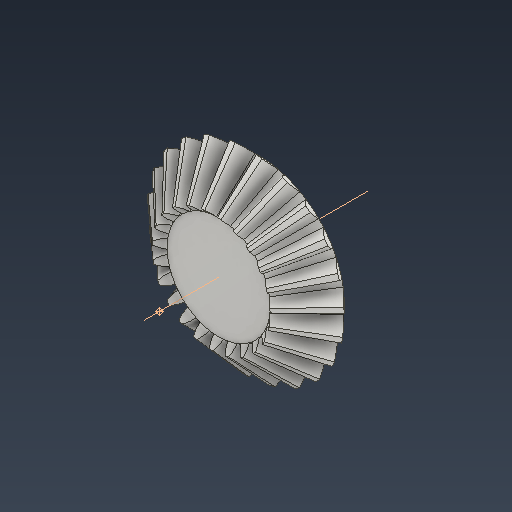
# Autodesk Inventor part: Kegelrad1
Saved by Autodesk Inventor 2021 (Build 250183000, 183)
## iProperties
Created: 2021-01-24
Part Number: Kegelrad1
Material: Steel, Mild
Document SubType Name: Modeling
Designer: laure
Categories: <?xml version="1.0" encoding="UTF-16"?> <MemberInstance><Categories><FamilyTemplate><FamilyTemplateParameter ValueType="xs:double" Id="1" ObjectReferenceKey="da_z" ObjectType="kUserParameterObject"/><FamilyTemplateParameter ValueType="xs:double" Id="2" ObjectReferenceKey="da_b" ObjectType="kUserParameterObject"/><FamilyTemplateParameter ValueType="xs:double" Id="3" ObjectReferenceKey="da_beta" ObjectType="kUserParameterObject"/><FamilyTemplateParameter ValueType="xs:double" Id="4" ObjectReferenceKey="da_dae" ObjectType="kUserParameterObject"/><FamilyTemplateParameter ValueType="xs:double" Id="5" ObjectReferenceKey="da_ve" ObjectType="kUserParameterObject"/><FamilyTemplateParameter ValueType="xs:double" Id="6" ObjectReferenceKey="da_omega" ObjectType="kUserParameterObject"/><FamilyTemplateParameter ValueType="xs:string" Id="7" ObjectReferenceKey="EAIAABAAAAAAHwAAAAAAAIAAAAAAAAAA" ObjectType="83914240" SubObjectId="SurfaceGeometry"/></FamilyTemplate><ParamToTemplateMap><ParamToTemplate CategoryParameter="//CategoryParameter[@InternalName='046C89C9-8512-4d59-83FE-43B91F4F132A']" TemplateParameter="1"/><ParamToTemplate CategoryParameter="//CategoryParameter[@InternalName='2552DF32-E462-4b46-AEBF-C6C7768E72AC']" TemplateParameter="2"/><ParamToTemplate CategoryParameter="//CategoryParameter[@InternalName='C9EE641D-15FC-4fae-A226-E94C4372FDD7']" TemplateParameter="3"/><ParamToTemplate><ParamToTemplate CategoryParameter="//CategoryParameter[@InternalName='00B6519A-459B-49c7-AD84-2E56D39A5744']" ConstantValue="0.000000"/></ParamToTemplate><ParamToTemplate><ParamToTemplate CategoryParameter="//CategoryParameter[@InternalName='04B31F0E-C7A6-4894-AA32-9629BEFACF47']" ConstantValue="1.000000"/></ParamToTemplate><ParamToTemplate><ParamToTemplate CategoryParameter="//CategoryParameter[@InternalName='43CBEC2E-7847-49e7-A936-2F7889FCB2D9']" ConstantValue="0.200000"/></ParamToTemplate><ParamToTemplate><ParamToTemplate CategoryParameter="//CategoryParameter[@InternalName='B1EFC894-105D-4ebd-86BF-FA20ED196853']" ConstantValue="0.300000"/></ParamToTemplate><ParamToTemplate><ParamToTemplate CategoryParameter="//CategoryParameter[@InternalName='51175063-3D10-4879-93E8-6246FE8B403D']" ConstantValue="2060000000.000000"/></ParamToTemplate><ParamToTemplate><ParamToTemplate CategoryParameter="//CategoryParameter[@InternalName='A3A52E27-4454-46a9-B0BD-C932399B70AF']" ConstantValue="0.300000"/></ParamToTemplate><ParamToTemplate CategoryParameter="//CategoryParameter[@InternalName='2A200944-5A8C-41ca-B96E-8520D2E510F1']" TemplateParameter="4"/><ParamToTemplate><ParamToTemplate CategoryParameter="//CategoryParameter[@InternalName='1A637F62-92C8-44bc-B81F-10802510B579']" ConstantValue="2.931322"/></ParamToTemplate><ParamToTemplate CategoryParameter="//CategoryParameter[@InternalName='B52DD4BE-6863-48fb-BF58-89EF6F9EC65C']" TemplateParameter="5"/><ParamToTemplate><ParamToTemplate CategoryParameter="//CategoryParameter[@InternalName='3956BFF2-84D2-457d-93C2-9B0613DEBA67']" ConstantValue="1.295862"/></ParamToTemplate><ParamToTemplate CategoryParameter="//CategoryParameter[@InternalName='739CFA02-461B-4bf8-8049-181FCAD8B28F']" TemplateParameter="6"/><ParamToTemplate><ParamToTemplate CategoryParameter="//CategoryParameter[@InternalName='A27E999F-E2CE-4481-8A2A-EBF499C4C3C5']" ConstantValue="0.000000"/></ParamToTemplate><ParamToTemplate><ParamToTemplate CategoryParameter="//CategoryParameter[@InternalName='9E1B4470-B2D3-4ff1-B813-535BB4CDF51A']" ConstantValue="3520000.000000"/></ParamToTemplate><ParamToTemplate><ParamToTemplate CategoryParameter="//CategoryParameter[@InternalName='F8452263-BFF6-458c-9FB1-07C4B99E95CD']" ConstantValue="11400000.000000"/></ParamToTemplate><ParamToTemplate><ParamToTemplate CategoryParameter="//CategoryParameter[@InternalName='3E3BB259-FD49-497f-8171-6EBC954A3479']" ConstantValue="2.000000"/></ParamToTemplate><ParamToTemplate CategoryParameter="//CategoryParameter[@InternalName='27C3BAF2-7550-4e4b-AE2C-0DB134B7D9B7']" TemplateParameter="7"/></ParamToTemplateMap><Category DisplayName="Gear" InternalName="DC85795E-93AB-48d5-8EEE-5A27447B64BD" Mnemonic="Gear"><CategoryParameter DisplayName="z" InternalName="046C89C9-8512-4d59-83FE-43B91F4F132A" Mnemonic="z"/><CategoryParameter DisplayName="b" InternalName="2552DF32-E462-4b46-AEBF-C6C7768E72AC" Mnemonic="b"/><CategoryParameter DisplayName="||b|" InternalName="C9EE641D-15FC-4fae-A226-E94C4372FDD7" Mnemonic="beta"/><CategoryParameter DisplayName="x" InternalName="00B6519A-459B-49c7-AD84-2E56D39A5744" Mnemonic="x"/><CategoryParameter DisplayName="a*" InternalName="04B31F0E-C7A6-4894-AA32-9629BEFACF47" Mnemonic="a"/><CategoryParameter DisplayName="c*" InternalName="43CBEC2E-7847-49e7-A936-2F7889FCB2D9" Mnemonic="c"/><CategoryParameter DisplayName="r|.f|*" InternalName="B1EFC894-105D-4ebd-86BF-FA20ED196853" Mnemonic="rf"/><CategoryParameter DisplayName="E" InternalName="51175063-3D10-4879-93E8-6246FE8B403D" Mnemonic="E"/><CategoryParameter DisplayName="||m|" InternalName="A3A52E27-4454-46a9-B0BD-C932399B70AF" Mnemonic="mi"/><Category DisplayName="BevelGear" InternalName="0C98F69A-0C2B-4791-B2FE-7691BB227E77" Mnemonic="BevelGear"><CategoryParameter DisplayName="d|.ae|" InternalName="2A200944-5A8C-41ca-B96E-8520D2E510F1" Mnemonic="dae"/><CategoryParameter DisplayName="d|.ai|" InternalName="1A637F62-92C8-44bc-B81F-10802510B579" Mnemonic="dai"/><CategoryParameter DisplayName="A|.e|" InternalName="B52DD4BE-6863-48fb-BF58-89EF6F9EC65C" Mnemonic="ve"/><CategoryParameter DisplayName="A|.i|" InternalName="3956BFF2-84D2-457d-93C2-9B0613DEBA67" Mnemonic="vi"/><CategoryParameter DisplayName="||S|" InternalName="739CFA02-461B-4bf8-8049-181FCAD8B28F" Mnemonic="omega"/><CategoryParameter DisplayName="x|.t|" InternalName="A27E999F-E2CE-4481-8A2A-EBF499C4C3C5" Mnemonic="xt"/><CategoryParameter DisplayName="||s||.Flim|" InternalName="9E1B4470-B2D3-4ff1-B813-535BB4CDF51A" Mnemonic="sFlim"/><CategoryParameter DisplayName="||s||.Hlim|" InternalName="F8452263-BFF6-458c-9FB1-07C4B99E95CD" Mnemonic="sHlim"/><CategoryParameter DisplayName="Typ" InternalName="3E3BB259-FD49-497f-8171-6EBC954A3479" Mnemonic="type"/><CategoryParameter DisplayName="PitchDiameter" InternalName="27C3BAF2-7550-4e4b-AE2C-0DB134B7D9B7" Mnemonic="IDS_PITCHDIAM"/></Category></Category></Categories></MemberInstance>
Mass: 60.9118 g
Surface Area: 34.3074 cm^2
Volume: 7.7496 cm^3
Density: 7.86 g/cm^3
Appearance: Steel
CustomPartVersion: 1
Author: laure
Autodesk Inventor part; units mm, degrees
ref_plane "Netzebene2" through (0, 0, 0) normal (0.9906859, 0.1361666, 0) x (0, 0, 1)
sketch "Skizze des Zahnradkörpers" plane through (0, 0, 0) normal (1, 0, 0) x (0, 1, 0)
  line L0 (0, 0) -> (21.302944, -24.697056) construction
  line L1 (21.302944, -24.697056) -> (24.414214, -21.585786)
  line L2 (24.414214, -21.585786) -> (0, 0) construction
  line L3 (23, -23) -> (0, 0) construction
  line L4 (12.788816, -14.826407) -> (14.656608, -12.958616)
  line L5 (21.302944, -24.697056) -> (12.788816, -14.826407)
  line L6 (24.414214, -21.585786) -> (14.656608, -12.958616)
  line L7 (0, -39.386751) -> (0, 6.564458)
  line L8 (0, -23) -> (24.414214, -23) construction
  dimension "d0" = 46
  dimension "d1" = 42.60589
  dimension "d2" = 48.82843
  dimension "d3" = 13
  dimension "d4" = 21.58579
  constraints: 16 end point, 4 point on line, 3 perpendicular, 2 collinear, 1 horizontal alignment, 1 vertical alignment
  measures "d0" diameter of L3.start L7
  measures "d1" diameter of L0.end L7
  measures "d2" diameter of L1.end L7
  measures "d3" distance between parallel lines of L1 L4
  measures "d4" vertical distance of L1.end L0.start
revolve "Zahnradkörper" add sketch "Skizze des Zahnradkörpers" angle 360 about axis through (0, 0, 0) along (0, 0, 1)
ref_plane "Zahnebene" through (0, 23, -23) normal (0, -0.7071068, 0.7071068) x (1, 0, 0)
sketch "Startskizze" plane through (0, 23, -23) normal (0, -0.7071068, 0.7071068) x (1, 0, 0)
  line L0 (0, -23.505131) -> (0, 10.644758)
  arc A0 (-0.779716, -2.928) -> (-3.579239, 3.140863) centre (-12.46349, -4.637511) ccw
  arc A1 (3.579239, 3.140863) -> (0.779716, -2.928) centre (12.46349, -4.637511) ccw
  line L1 (-0.779716, -2.928) -> (0.779716, -2.928)
  arc A2 (3.579239, 3.140863) -> (-3.579239, 3.140863) centre (0, -32.526912) ccw
  dimension "d7" = 11.80818
  dimension "d8" = 12.46349
  dimension "d9" = 27.8894
  dimension "d57" = 35.84691
  dimension "d58" = 29.59891
  constraints: 6 point on circle, 3 centre point, 3 symmetric about line, 2 end point, 1 coincident, 1 perpendicular, 1 other
  measures "d7" radius of A0
  measures "d8" horizontal distance of point (0, -32.527) A0.centre
  measures "d9" vertical distance of point (0, -32.527) A0.centre
  measures "d57" radius of A2
  measures "d58" distance from line of A2.centre L1
ref_plane "Endebene" through (0, 13.652048, -13.652048) normal (0, -0.7071068, 0.7071068) x (1, 0, 0)
sketch "Endskizze" plane through (0, 13.652048, -13.652048) normal (0, -0.7071068, 0.7071068) x (1, 0, 0)
  line L0 (0, -15.35404) -> (0, 6.953444)
  arc A0 (-0.462814, -1.737965) -> (-2.124519, 1.864313) centre (-7.39792, -2.752675) ccw
  arc A1 (2.124519, 1.864313) -> (0.462814, -1.737965) centre (7.39792, -2.752675) ccw
  line L1 (-0.462814, -1.737965) -> (0.462814, -1.737965)
  arc A2 (2.124519, 1.864313) -> (-2.124519, 1.864313) centre (0, -19.306912) ccw
  dimension "d12" = 7.00895
  dimension "d15" = 7.39792
  dimension "d16" = 16.55424
  dimension "d59" = 21.27756
  dimension "d60" = 17.56895
  constraints: 6 point on circle, 3 centre point, 3 symmetric about line, 2 end point, 1 coincident, 1 other
  measures "d12" radius of A0
  measures "d15" horizontal distance of A0.centre point (0, -19.307)
  measures "d16" vertical distance of A0.centre point (0, -19.307)
  measures "d59" radius of A2
  measures "d60" distance from line of A2.centre L1
loft "Loft" cut profiles "Startskizze", "Endskizze"
pattern_circular "Circular Pattern" count 23 over 360 about axis through (0, 0, 0) along (0, 0, 1) of "Loft"
sketch3d "3D-Skizze rechts"
ref_plane "Endebene rechts" through (-3.528811, 13.188098, -13.652048) normal (0.1827745, -0.6830765, 0.7071068) x (0.966016, 0.2584821, 0)
sketch "Endskizze rechts" plane through (-3.528811, 13.188098, -13.652048) normal (0.1827745, -0.6830765, 0.7071068) x (0.966016, 0.2584821, 0)
  arc A0 (-0.462814, -1.737965) -> (-2.124519, 1.864313) centre (-7.39792, -2.752675) ccw
  line L0 (0, -27.178838) -> (0, 11.63858)
  arc A1 (2.124519, 1.864313) -> (0.462814, -1.737965) centre (7.39792, -2.752675) ccw
  line L1 (-0.462814, -1.737965) -> (0.462814, -1.737965)
  arc A2 (2.124519, 1.864313) -> (-2.124519, 1.864313) centre (0, -19.306912) ccw
  dimension "d70" = 7.39792
  dimension "d71" = 16.55424
  dimension "d72" = 7.00895
  dimension "d73" = 17.56895
  dimension "d74" = 21.27756
  constraints: 6 point on circle, 3 centre point, 3 symmetric about line, 2 end point, 1 coincident, 1 perpendicular, 1 other
  measures "d70" horizontal distance of A2.centre A0.centre
  measures "d71" vertical distance of point (0, -19.307) A0.centre
  measures "d72" radius of A0
  measures "d73" distance from line of point (0, -19.307) L1
  measures "d74" radius of A2
feature "Erhebung rechts" [suppressed]
pattern_circular "Runde Anordnung rechts" [suppressed]
sketch3d "3D-Skizze links"
ref_plane "Endebene links" through (3.526465, 13.188098, -13.651163) normal (-0.182663, -0.6831138, 0.7070996) x (0.9660589, -0.2583218, 0)
sketch "Endskizze links" plane through (3.526465, 13.188098, -13.651163) normal (-0.182663, -0.6831138, 0.7070996) x (0.9660589, -0.2583218, 0)
  line L0 (0, -32.200608) -> (0, 15.177885)
  arc A0 (-0.462814, -1.738162) -> (-2.124519, 1.864116) centre (-7.39792, -2.752872) ccw
  arc A1 (2.124519, 1.864116) -> (0.462814, -1.738162) centre (7.39792, -2.752872) ccw
  line L1 (-0.462814, -1.738162) -> (0.462814, -1.738162)
  ellipse E0 centre (0, -9.163219) end of major axis (14.656608, -9.163219) minor radius 10.363681
  arc A2 (2.124519, 1.864116) -> (-2.124519, 1.864116) centre (0, -19.307109) ccw
  dimension "d56" = 10.36368
  dimension "d30" = 7.00895
  dimension "d31" = 7.39792
  dimension "d32" = 16.55424
  dimension "d61" = 21.27756
  dimension "d62" = 17.56895
  constraints: 6 point on circle, 3 centre point, 3 symmetric about line, 2 end point, 1 coincident, 2 other
  measures "d30" radius of A0
  measures "d31" horizontal distance of point (0, -19.307) A0.centre
  measures "d32" vertical distance of A0.centre point (0, -19.307)
  measures "d61" radius of A2
  measures "d62" distance from line of point (0, -19.307) L1
feature "Erhebung links" [suppressed]
pattern_circular "Runde Anordnung links" [suppressed]
sketch "Körperskizze" plane through (0, 0, 0) normal (1, 0, 0) x (0, 1, 0)
  line L0 (0, -35.037536) -> (0, -19.530831)
  line L1 (21.302944, -24.697056) -> (12.788816, -14.826407)
  line L2 (12.788816, -14.826407) -> (0, -14.826407)
  line L3 (21.302944, -24.697056) -> (0, -24.697056)
  constraints: 4 end point, 2 perpendicular, 2 point on line
sketch "Körperskizze outline for Festkörper" plane through (0, 0, 0) normal (1, 0, 0) x (0, 1, 0)
  line L0 (0, -24.697056) -> (21.302944, -24.697056)
  line L1 (0, -14.826407) -> (0, -24.697056)
  line L2 (12.788816, -14.826407) -> (0, -14.826407)
  line L3 (21.302944, -24.697056) -> (12.788816, -14.826407)
revolve "Festkörper" add sketch "Körperskizze outline for Festkörper" angle 360 about axis through (0, 0, 0) along (0, 0, 1)
sketch "Sketch6" plane through (0, 0, 0) normal (1, 0, 0) x (0, 1, 0)
  line L0 (23, -23) -> (0, 0)
  line L1 (0, -37.799919) -> (0, 6.299986)
surface revolve "Flankendurchmesser" sketch "Sketch6" angle 360 about axis through (0, 0, 0) along (0, 0, 1) shown no curves L0
equation "\"d0\" = da_de"
equation "\"d1\" = da_dfe"
equation "\"d2\" = da_dae"
equation "\"d3\" = da_b"
equation "\"d4\" = da_ve"
equation "\"d7\" = fd_rr"
equation "\"d8\" = fd_x"
equation "\"d9\" = fd_y"
equation "\"d57\" = 0.5 * fd_dva + 0.3 * da_he"
equation "\"d58\" = 0.5 * fd_dva - 1.12 * da_he"
equation "\"da_teethtype\" = 0"
equation "\"da_b\" = 13"
equation "\"da_de\" = 46"
equation "\"da_dae\" = 48.82843"
equation "\"da_dfe\" = 42.60589"
equation "\"da_le\" = 32.52691"
equation "\"da_omega\" = 90deg"
equation "\"da_beta\" = 0"
equation "\"da_delta\" = 45deg"
equation "\"da_alpha\" = 20deg"
equation "\"da_he\" = 4.4"
equation "\"da_ve\" = 21.58579"
equation "\"da_zv\" = 32.526912"
equation "\"fd_loft\" = da_b + 0.05 * da_he"
equation "\"fd_x\" = fd_x1 + fd_x2"
equation "\"fd_y\" = fd_y1 - fd_y2"
equation "\"fd_dd\" = fd_dva - 0.8 * da_he"
equation "\"da_dvw\" = 65.05382"
equation "\"d11\" = fd_loft"
equation "\"da_dm\" = 36.80761"
equation "\"da_x\" = 0"
equation "\"da_m\" = 2"
equation "\"d50\" = da_omega"
equation "\"fd_rr\" = 11.808175"
equation "\"fd_dva\" = 69.053824"
equation "\"fd_x1\" = 1.587619"
equation "\"fd_x2\" = 10.875871"
equation "\"fd_y1\" = 32.488143"
equation "\"fd_y2\" = 4.598742"
body "Solid1"
body "Srf1"
